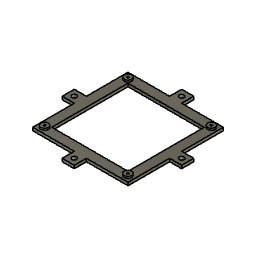
PCB_Mounting (Autodesk Fusion 360 design; units mm, degrees)
Autodesk Fusion 360 part; units mm, degrees
sketch "Sketch1" plane through (0, 0, 0) normal (0, 0, 1) x (1, 0, 0) in component "Bracket"
  line L0 (-40, 40) -> (40, 40)
  line L1 (40, 40) -> (40, -40)
  line L2 (40, -40) -> (-40, -40)
  line L3 (-40, -40) -> (-40, 40)
  line L4 (-50, 50) -> (50, 50)
  line L5 (50, 50) -> (50, -50)
  line L6 (50, -50) -> (-50, -50)
  line L7 (-50, -50) -> (-50, 50)
  circle A0 centre (-43.75, 43.75) radius 1
  circle A1 centre (-43.75, -43.75) radius 1
  circle A2 centre (43.75, -43.75) radius 1
  circle A3 centre (43.75, 43.75) radius 1
  line L8 (-6.35, 50) -> (-6.35, 62.7)
  line L9 (-6.35, 62.7) -> (6.35, 62.7)
  line L10 (6.35, 62.7) -> (6.35, 50)
  line L11 (-50, 6.35) -> (-62.7, 6.35)
  line L12 (-62.7, 6.35) -> (-62.7, -6.35)
  line L13 (-62.7, -6.35) -> (-50, -6.35)
  line L14 (-6.35, -50) -> (-6.35, -62.7)
  line L15 (-6.35, -62.7) -> (6.35, -62.7)
  line L16 (6.35, -62.7) -> (6.35, -50)
  line L17 (50, 6.35) -> (62.7, 6.35)
  line L18 (62.7, 6.35) -> (62.7, -6.35)
  line L19 (62.7, -6.35) -> (50, -6.35)
  circle A4 centre (56.35, 0) radius 2.5
  circle A5 centre (0, 56.35) radius 2.5
  circle A6 centre (-56.35, 0) radius 2.5
  circle A7 centre (0, -56.35) radius 2.5
  circle A8 centre (43.75, 43.75) radius 4
  circle A9 centre (-43.75, 43.75) radius 4
  circle A10 centre (-43.75, -43.75) radius 4
  circle A11 centre (43.75, -43.75) radius 4
  dimension "d1" = 80
  dimension "d2" = 80
  dimension "d3" = 100
  dimension "d4" = 100
  dimension "d5" = 40
  dimension "d6" = 50
  dimension "d7" = 40
  dimension "d8" = 50
  dimension "d11" = 2
  dimension "d12" = 2
  dimension "d13" = 2
  dimension "d14" = 2
  dimension "d15" = 87.5
  dimension "d16" = 87.5
  dimension "d17" = 43.75
  dimension "d18" = 43.75
  dimension "d19" = 12.7
  dimension "d20" = 12.7
  dimension "d21" = 6.35
  dimension "d22" = 12.7
  dimension "d23" = 12.7
  dimension "d24" = 6.35
  dimension "d25" = 12.7
  dimension "d26" = 12.7
  dimension "d27" = 6.35
  dimension "d28" = 12.7
  dimension "d29" = 12.7
  dimension "d30" = 6.35
  dimension "d31" = 5
  dimension "d32" = 6.35
  dimension "d33" = 6.35
  dimension "d34" = 5
  dimension "d35" = 6.35
  dimension "d36" = 6.35
  dimension "d37" = 5
  dimension "d38" = 6.35
  dimension "d39" = 6.35
  dimension "d40" = 5
  dimension "d41" = 6.35
  dimension "d42" = 6.35
  dimension "d43" = 8
  dimension "d44" = 8
  dimension "d45" = 8
  dimension "d46" = 8
  constraint horizontal L0
  constraint vertical L1
  constraint horizontal L2
  constraint vertical L3
  constraint horizontal L4
  constraint vertical L5
  constraint horizontal L6
  constraint vertical L7
  constraint horizontal A1.centre A2.centre
  constraint vertical A2.centre A3.centre
  constraint horizontal A0.centre A3.centre
  constraint vertical A0.centre A1.centre
  constraint coincident L4 L8.start
  constraint perpendicular L4 L8
  constraint perpendicular L8 L9
  constraint coincident L4 L10.end
  constraint perpendicular L4 L10
  constraint coincident L7 L11.start
  constraint perpendicular L7 L11
  constraint perpendicular L11 L12
  constraint coincident L7 L13.end
  constraint perpendicular L7 L13
  constraint coincident L6 L14.start
  constraint perpendicular L6 L14
  constraint perpendicular L14 L15
  constraint coincident L6 L16.end
  constraint perpendicular L6 L16
  constraint coincident L5 L17.start
  constraint perpendicular L5 L17
  constraint perpendicular L0 L18
  constraint coincident L5 L19.end
  constraint perpendicular L5 L19
  constraint concentric A3 A8
  constraint concentric A0 A9
  constraint concentric A1 A10
  constraint concentric A2 A11
  measures "d1" distance of L0.start L0.end
  measures "d2" distance of L0.start L2.end
  measures "d3" distance of L4.start L4.end
  measures "d4" distance of L4.start L6.end
  measures "d5" distance of origin L0
  measures "d6" distance of origin L4
  measures "d7" distance of origin L1
  measures "d8" distance of origin L5
  measures "d11" diameter of A0
  measures "d12" diameter of A1
  measures "d13" diameter of A2
  measures "d14" diameter of A3
  measures "d15" horizontal distance of A0.centre A3.centre
  measures "d16" vertical distance of A0.centre A1.centre
  measures "d17" horizontal distance of origin A3.centre
  measures "d18" vertical distance of origin A3.centre
  measures "d19" distance of L8.end L9.end
  measures "d20" distance of L9.end L10.end
  measures "d21" distance of origin L10
  measures "d22" distance of L11.end L12.end
  measures "d23" distance of L11.start L11.end
  measures "d24" vertical distance of origin L11.start
  measures "d25" distance of L15.end L16.end
  measures "d26" distance of L14.end L15.end
  measures "d27" distance of origin L16
  measures "d28" distance of L17.end L18.end
  measures "d29" distance of L17.start L17.end
  measures "d30" distance of origin L17
  measures "d31" diameter of A4
  measures "d32" distance of L19 A4.centre
  measures "d33" distance of L18 A4.centre
  measures "d34" diameter of A5
  measures "d35" distance of L9 A5.centre
  measures "d36" distance of L8 A5.centre
  measures "d37" diameter of A6
  measures "d38" distance of L11 A6.centre
  measures "d39" distance of L12 A6.centre
  measures "d40" diameter of A7
  measures "d41" distance of L16 A7.centre
  measures "d42" distance of L15 A7.centre
  measures "d43" diameter of A8
  measures "d44" diameter of A9
  measures "d45" diameter of A10
  measures "d46" diameter of A11
extrude "Extrude1" add sketch "Sketch1" along normal blind 3.175 contours L4 L5 L6 L7 | L4 L8 L9 L10 | L7 L11 L12 L13 | L5 L17 L18 L19 | L6 L14 L15 L16 in component "Bracket"
extrude "Extrude2" add sketch "Sketch1" along normal blind 5 contours A8 | A9 | A10 | A11 in component "Bracket"
component "Bracket" placed x (1, 0, 0) y (0, 1, 0) z (0, 0, 1) at (0, 0, 0)
equation "d5 = d2 / 2"
equation "d6 = d4 / 2"
equation "d7 = d1 / 2"
equation "d8 = d3 / 2"
equation "d17 = d15 / 2"
equation "d18 = d16 / 2"
